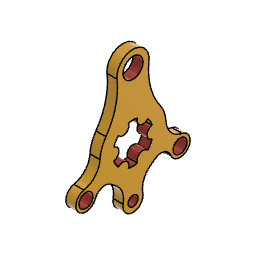
EXP-01_ (Autodesk Fusion 360 design; units mm, degrees)
Autodesk Fusion 360 part; units mm, degrees
sketch "Sketch1" plane through (0, 0, 0) normal (1, 0, 0) x (0, 1, 0)
  line L0 (0, 90) -> (0, -120)
  circle A0 centre (0, 65) radius 10
  circle A1 centre (-47, -26) radius 7
  circle A2 centre (0, -50) radius 5
  arc A3 (-27.0298, 18.9312) -> (-15.8903, 63.1292) centre (-79.4513, 55.6462) ccw
  arc A4 (-48.9633, -16.1946) -> (-32.9314, 2.127) centre (-52.8898, 3.4162) ccw
  arc A5 (-21.5665, -24.9777) -> (-37.5509, -29.2733) centre (-28.1018, -32.5467) ccw
  arc A6 (-9.804, -48.03) -> (-18.3132, -27.4523) centre (-29.4121, -44.09) ccw
  circle A7 centre (0, 65) radius 10
  arc A8 (15.8903, 63.1292) -> (27.0298, 18.9312) centre (79.4513, 55.6462) ccw
  arc A9 (32.9314, 2.127) -> (48.9633, -16.1946) centre (52.8898, 3.4162) ccw
  circle A10 centre (47, -26) radius 7
  arc A11 (18.3132, -27.4523) -> (9.804, -48.03) centre (29.4121, -44.09) ccw
  arc A12 (37.5509, -29.2733) -> (21.5665, -24.9777) centre (28.1018, -32.5467) ccw
  circle A13 centre (0, -50) radius 5
  arc A14 (15.8903, 63.1292) -> (-15.8903, 63.1292) centre (0, 65) ccw
  arc A15 (15.8903, 63.1292) -> (-15.8903, 63.1292) centre (0, 65) ccw
  arc A16 (-27.0298, 18.9312) -> (-32.9314, 2.127) centre (0, 0) ccw
  arc A17 (-27.0298, 18.9312) -> (-32.9314, 2.127) centre (0, 0) ccw
  arc A18 (-21.5665, -24.9777) -> (-18.3132, -27.4523) centre (0, 0) ccw
  arc A19 (-21.5665, -24.9777) -> (-18.3132, -27.4523) centre (0, 0) ccw
  arc A20 (18.3132, -27.4523) -> (21.5665, -24.9777) centre (0, 0) ccw
  arc A21 (32.9314, 2.127) -> (27.0298, 18.9312) centre (0, 0) ccw
  arc A22 (18.3132, -27.4523) -> (21.5665, -24.9777) centre (0, 0) ccw
  arc A23 (32.9314, 2.127) -> (27.0298, 18.9312) centre (0, 0) ccw
  arc A24 (-48.9633, -16.1946) -> (-37.5509, -29.2733) centre (-47, -26) ccw
  arc A25 (-9.804, -48.03) -> (9.804, -48.03) centre (0, -50) ccw
  arc A26 (-9.804, -48.03) -> (9.804, -48.03) centre (0, -50) ccw
  arc A27 (37.5509, -29.2733) -> (48.9633, -16.1946) centre (47, -26) ccw
  arc A28 (-19.1, -5.9321) -> (-19.1, 5.9321) centre (-20, 0) ccw
  arc A29 (-4.4126, -19.5071) -> (-14.6874, -13.575) centre (-10, -17.3205) ccw
  arc A30 (14.6874, -13.575) -> (4.4126, -19.5071) centre (10, -17.3205) ccw
  arc A31 (19.1, 5.9321) -> (19.1, -5.9321) centre (20, 0) ccw
  arc A32 (4.4126, 19.5071) -> (14.6874, 13.575) centre (10, 17.3205) ccw
  arc A33 (-14.6874, 13.575) -> (-4.4126, 19.5071) centre (-10, 17.3205) ccw
  arc A34 (-14.6874, 13.575) -> (-19.1, 5.9321) centre (0, 0) ccw
  arc A35 (-14.6874, 13.575) -> (-19.1, 5.9321) centre (0, 0) ccw
  arc A36 (4.4126, 19.5071) -> (-4.4126, 19.5071) centre (0, 0) ccw
  arc A37 (4.4126, 19.5071) -> (-4.4126, 19.5071) centre (0, 0) ccw
  arc A38 (19.1, 5.9321) -> (14.6874, 13.575) centre (0, 0) ccw
  arc A39 (19.1, 5.9321) -> (14.6874, 13.575) centre (0, 0) ccw
  arc A40 (14.6874, -13.575) -> (19.1, -5.9321) centre (0, 0) ccw
  arc A41 (14.6874, -13.575) -> (19.1, -5.9321) centre (0, 0) ccw
  arc A42 (-19.1, -5.9321) -> (-14.6874, -13.575) centre (0, 0) ccw
  arc A43 (-4.4126, -19.5071) -> (4.4126, -19.5071) centre (0, 0) ccw
  arc A44 (-19.1, -5.9321) -> (-14.6874, -13.575) centre (0, 0) ccw
  arc A45 (-4.4126, -19.5071) -> (4.4126, -19.5071) centre (0, 0) ccw
  dimension "d8" = 65
  dimension "d9" = 26
  dimension "d10" = 24
  dimension "d11" = 47
  dimension "d12" = 64
  dimension "d13" = 20
  dimension "d14" = 10
  dimension "d15" = 20
  dimension "d18" = 360
  dimension "d21" = 6
  constraint vertical L0
  constraint coincident L0 A0.centre
  constraint concentric A0 A14
  constraint coincident A16.centre A17.centre
  constraint concentric A1 A24
  constraint coincident L0 A2.centre
  constraint concentric A2 A26
  constraint tangent A3 A14
  constraint tangent A3 A16
  constraint tangent A4 A24
  constraint tangent A4 A16
  constraint tangent A5 A24
  constraint coincident A5.start A16
  constraint tangent A5 A16
  constraint tangent A6 A16
  constraint coincident A6.end A16
  constraint tangent A6 A26
  constraint symmetric L0 A0 A7
  constraint symmetric L0 A14 A15
  constraint symmetric L0 A42 A44
  constraint symmetric L0 A16 A17
  constraint symmetric L0 A24 A27
  constraint symmetric L0 A1 A10
  constraint symmetric L0 A25 A26
  constraint symmetric L0 A2 A13
  constraint symmetric L0 A3.end A8.start
  constraint symmetric L0 A3.start A8.end
  constraint symmetric L0 A3 A8
  constraint symmetric L0 A4.end A9.start
  constraint symmetric L0 A4.start A9.end
  constraint symmetric L0 A4 A9
  constraint symmetric L0 A5.end A12.start
  constraint symmetric L0 A5.start A12.end
  constraint symmetric L0 A5 A12
  constraint symmetric L0 A6.start A11.end
  constraint symmetric L0 A6.end A11.start
  constraint symmetric L0 A6 A11
  constraint concentric A16 A19
  constraint concentric A17 A18
  constraint concentric A18 A20
  constraint concentric A19 A22
  constraint concentric A20 A21
  constraint concentric A22 A23
  constraint coincident A28.centre A42
  constraint concentric A34 A42
  constraint concentric A35 A44
  constraint concentric A36 A42
  constraint concentric A37 A44
  constraint concentric A38 A44
  constraint concentric A39 A42
  constraint concentric A40 A44
  constraint concentric A41 A42
  constraint concentric A42 A43
  constraint concentric A44 A45
  measures "d8" distance of A0.centre A16.centre
  measures "d9" vertical distance of A16.centre A1.centre
  measures "d10" vertical distance of A1.centre A2.centre
  measures "d11" horizontal distance of A1.centre A2.centre
  measures "d12" radius of A3
  measures "d13" radius of A4
  measures "d14" radius of A5
  measures "d15" radius of A6
  measures "d21" radius of A33
extrude "Extrude1" add sketch "Sketch1" along normal blind 10 contours L0 A0 A2 A7 A8 A9 A11 A12 A13 A14 A15 A20 A21 A22 A23 A25 A26 A27 A30 A31 A32 A36 A37 A38 A39 A40 A41 A43 A45 | L0 A0 A2 A3 A4 A5 A6 A7 A13 A14 A15 A16 A17 A18 A19 A24 A25 A26 A28 A29 A33 A34 A35 A36 A37 A42 A43 A44 A45
